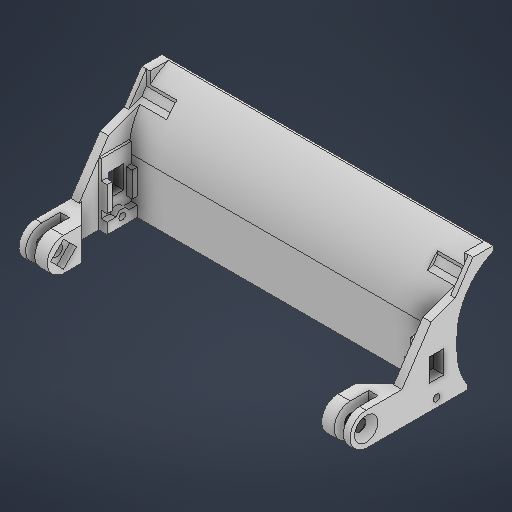
# Autodesk Inventor part: body-main
Saved by Autodesk Inventor 2025 (Build 290162000, 162)
## iProperties
Created: 2025-03-21
Part Number: body-main
Material: Všeobecné
Document SubType Name: Modeling
Designer: Simak
Density: 1 g/cm^3
Appearance: Výchozí
Author: Simak
Autodesk Inventor part; units mm, degrees
ref_plane "YZ Plane" through (0, 0, 0) normal (1, 0, 0) x (0, 1, 0)
ref_plane "XZ Plane" through (0, 0, 0) normal (0, 1, 0) x (-1, 0, 0)
ref_plane "XY Plane" through (0, 0, 0) normal (0, 0, 1) x (1, 0, 0)
sketch "Náčrt1" plane through (0, 0, 0) normal (1, 0, 0) x (0, 1, 0)
  circle A0 centre (13.5, 0) radius 16.5 construction
  circle A1 centre (15.5, 0) radius 16.5 construction
  circle A2 centre (11.5, 0) radius 16.5 construction
  line L0 (15.5, 16.5) -> (11.5, 16.5) construction
  line L1 (15.5, -16.5) -> (11.5, -16.5) construction
  circle A3 centre (5, 45.139) radius 5
  line L2 (0, 0) -> (0, 45.139)
  line L3 (10, 34.353) -> (22.9651, 25.7096)
  line L4 (10, 34.353) -> (10, 45.139)
  line L5 (22.9651, 25.7096) -> (27.5, 13.25)
  line L6 (27.5, 13.25) -> (33.5, 13.25)
  line L7 (33.5, 13.25) -> (25.5777, 18.5315)
  line L8 (33.5, 13.25) -> (33.5, 7.1937)
  line L9 (29, 13.25) -> (27.0194, 14.5704)
  arc A4 (13.5, -17.8885) -> (15.5, 18) centre (15.5, 0) ccw
  arc A5 (11.5, 18) -> (13.5, -17.8885) centre (11.5, 0) ccw
  line L10 (15.5, 18) -> (11.5, 18)
  line L11 (1.5, 14.9666) -> (0, 14.9666)
  line L12 (33.5, 7.1937) -> (32, 7.1937)
  arc A6 (13.5, -19.4977) -> (15.5, 19.6) centre (15.5, 0) ccw
  arc A7 (11.5, 19.6) -> (13.5, -19.4977) centre (11.5, 0) ccw
  line L13 (11.5, 19.6) -> (15.5, 19.6)
  line L14 (21.6, 28.6) -> (0, 28.6) construction
  line L15 (0, 28.6) -> (0, 19.6)
  line L16 (0, 19.6) -> (21.6, 19.6)
  line L17 (21.6, 19.6) -> (21.6, 28.6) construction
  line L18 (35.6, 21.5) -> (34, 21.5) construction
  line L19 (34, 21.5) -> (34, -16) construction
  line L20 (34, -16) -> (35.6, -16) construction
  line L21 (35.6, -16) -> (35.6, 21.5) construction
  line L22 (35.6, 17.75) -> (34, 17.75) construction
  line L23 (33.2196, 14.55) -> (26.5242, 14.55) construction
  line L24 (10, 39.639) -> (0, 39.639)
  line L25 (10, 34.353) -> (9.85, 34.453)
  line L26 (9.85, 34.453) -> (9.85, 39.639)
  point P0 (26.3917, 16.2951)
  point P1 (33.5, 7.7563)
  point P2 (29.9429, 13.25)
  dimension "d0" = 33
  dimension "d1" = 2
  dimension "d2" = 2
  dimension "d3" = 13.5
  dimension "d4" = 10
  dimension "d5" = 45.139
  dimension "d6" = 10.786
  dimension "d8" = 123.69
  dimension "d10" = 13.25
  dimension "d11" = 33.5
  dimension "d12" = 6
  dimension "d16" = 1.5
  dimension "d17" = 36
  dimension "d18" = 36
  dimension "d19" = 1.5
  dimension "d20" = 1.5
  dimension "d21" = 1.6
  dimension "d23" = 9
  dimension "d24" = 21.6
  dimension "d25" = 0.5
  dimension "d26" = 1.6
  dimension "d27" = 37.5
  dimension "d28" = 3.75
  dimension "d29" = 20.5
  dimension "d30" = 3.2
  dimension "d41" = 5.5
  dimension "d45" = 9.85
  dimension "d86" = 70
  constraints: 54 end point, 17 point on circle, 11 point on line, 8 centre point, 8 perpendicular, 7 horizontal, 5 parallel, 5 tangent, 3 horizontal alignment, 3 vertical, 2 coincident, 2 collinear, 2 equal radius, 2 other
  measures "d0" diameter of A0
  measures "d1" distance of A0.centre A1.centre
  measures "d2" distance of A0.centre A2.centre
  measures "d3" distance of A0.centre L2.start
  measures "d4" diameter of A3
  measures "d5" vertical distance of A3.centre A0.centre
  measures "d6" vertical distance of A3.centre L3.start
  measures "d8" angle of L4 L3
  measures "d10" distance from line of A1.centre L6
  measures "d11" distance from line of L2 L6.end
  measures "d12" distance of L5.end L6.end
  measures "d16" distance of L5.end L9.start
  measures "d17" diameter of A4
  measures "d18" diameter of A5
  measures "d19" distance of L11.start L11.end
  measures "d20" distance of L8.end L12.end
  measures "d21" radial gap between concentric circles of A4 A6
  measures "d23" distance of L16.end L14.start
  measures "d24" distance of L14.start L14.end
  measures "d25" distance between parallel lines of L20 L1
  measures "d26" distance of L19.end L20.end
  measures "d27" distance of L20.end L18.start
  measures "d28" distance between parallel lines of L18 L22
  measures "d29" distance from line of L19 A0.centre
  measures "d30" distance between parallel lines of L22 L23
  measures "d41" distance from line of A3.centre L24
  measures "d45" distance between parallel lines of L2 L26
  measures "d86" angle of L6 L5
extrude "Vysunutí1" add sketch "Náčrt1" against normal blind 2.5 contours L24 L26 L25 L3 L5 A6 L13 L16 L2 | L16 A7 L2 | A7 L13 A6 L5 A4 L10 A5 L11 L2 | L8 A6 L6 | L9 L6 A4 L5 | A6 L8 L12 A4 L6
extrude "Vysunutí3" add sketch "Náčrt1" against normal blind 49.5 contours L16 A7 L2 | A7 L13 A6 L5 A4 L10 A5 L11 L2 | A6 L6 L9 L5 | L9 L6 A4 L5 | A6 L8 L12 A4 L6
extrude "Vysunutí4" cut sketch "Náčrt1" against normal blind 10.5 contours A6 L6 L9 L5
extrude "Vysunutí5" add sketch "Náčrt1" against normal blind 1.35 contours L7 L6 A6 L5 | A6 L6 L9 L5
sketch "Náčrt2" plane through (0, 0, 0) normal (1, 0, 0) x (0, 0, -1)
  circle A0 centre (-45.139, 5) radius 4.85
  line L0 (-46.7978, 0.4425) -> (-45.5821, 0)
  line L1 (-19.6, 0) -> (-39.639, 0) projected
  line L2 (-39.639, 0) -> (-45.5821, 0)
  line L3 (-39.639, 9.85) -> (-39.639, 0) projected
  line L4 (-39.639, 9.85) -> (-45.139, 9.85)
  line L5 (-45.139, 8.8891) -> (-49.0281, 5)
  line L6 (-49.0281, 5) -> (-45.139, 1.1109)
  line L7 (-45.139, 1.1109) -> (-41.2499, 5)
  line L8 (-41.2499, 5) -> (-45.139, 8.8891)
  line L9 (-45.139, 8.8891) -> (-45.139, 5) construction
  line L10 (-45.139, 5) -> (-41.2499, 5) construction
  line L11 (-45.139, 5) -> (-45.139, 1.1109) construction
  point P0 (0, 0)
  dimension "d42" = 9.7
  dimension "d44" = 20
  dimension "d47" = 5.5
  constraints: 20 end point, 5 equal length, 4 perpendicular, 2 point on circle, 2 tangent, 1 centre point, 1 coincident, 1 collinear, 1 vertical
  measures "d42" diameter of A0
  measures "d44" angle of L2 L0
  measures "d47" distance of L7.end L5.start
extrude "Vysunutí6" add sketch "Náčrt2" against normal blind 8.5 contours A0 | A0 L4 L3 L2 L0 | L8 L7 L6 L5
sketch "Náčrt3" plane through (0, 0, 0) normal (1, 0, 0) x (0, 0, -1)
  arc A0 (-45.139, 9.85) -> (-46.7978, 0.4425) centre (-45.139, 5) ccw construction
  point P0 (0, 0)
  constraints: 1 coincident
hole "Díra1" at (0, 5, 45.139) direction (-1, 0, 0) diameter 3.4 end through all countersink diameter 7 countersink angle 90
sketch "Náčrt4" plane through (-8.5, 0, 0) normal (-1, 0, 0) x (0, 0, 1)
  line L0 (45.139, 1.1109) -> (41.2499, 5) projected
  line L1 (41.2499, 5) -> (45.139, 8.8891) projected
  line L2 (45.139, 8.8891) -> (49.0281, 5) projected
  line L3 (49.0281, 5) -> (45.139, 1.1109) projected
  point P0 (0, 0)
extrude "Vysunutí7" cut sketch "Náčrt4" against normal blind 2
sketch "Náčrt5" plane through (-2.5, 9.85, 34.453) normal (0, 1, 0) x (1, 0, 0)
  line L0 (2.5, -15.536) -> (-6, -15.536) projected
  line L1 (0.5, -15.536) -> (0.5, -5.186)
  line L2 (0.7, -12.386) -> (0.7, -8.986) projected
  line L3 (0.5, -5.186) -> (-2.25, -5.186)
  line L4 (-2.25, -5.186) -> (-2.25, -15.536)
  line L5 (2.5, 0) -> (2.5, -10.686) projected
  line L6 (2.5, -10.686) -> (-6, -10.686) projected
  line L7 (-6, -10.686) -> (-6, -5.186) projected
  line L8 (-6, -5.186) -> (0, 0.814)
  line L9 (0, 0) -> (0, 8.7433) projected
  line L10 (0, -5.186) -> (-6, -5.186) projected
  line L11 (0, -5.186) -> (0, 0) projected
  point P0 (2.5, 34.453)
  dimension "d59" = 2
  dimension "d60" = 2.75
  dimension "d61" = 5.5
  dimension "d62" = 45
  constraints: 8 end point, 2 perpendicular, 2 point on line, 1 parallel
  measures "d59" distance between parallel lines of L5 L1
  measures "d60" distance of L1.end L3.end
  measures "d61" distance between parallel lines of L3 L6
  measures "d62" angle of L10 L8
extrude "Vysunutí8" add sketch "Náčrt5" against normal up to surface (9.85 mm away) contours L10 L8 L9 L11 L3
extrude "Vysunutí9" cut sketch "Náčrt5" against normal through all contours L0 L4 L6 L1 | L6 L4 L3 L1
sketch "Náčrt6" plane through (-2.5, 0, 0) normal (-1, 0, 0) x (0, 0, 1)
  line L0 (19.6, 21.6) -> (28.6, 21.6) projected
  line L1 (28.6, 21.6) -> (28.6, 0) projected
  line L2 (19.6, 0) -> (19.6, 21.6) projected
  line L3 (19.6, 0) -> (33.639, 0) projected
  circle A0 centre (24.1, 2.54) radius 1
  line L4 (22.9, 13.2) -> (25.3, 13.2)
  line L5 (25.3, 13.2) -> (25.3, 8.4)
  line L6 (25.3, 8.4) -> (22.9, 8.4)
  line L7 (22.9, 8.4) -> (22.9, 13.2)
  line L8 (21.9, 14.2) -> (26.3, 14.2)
  line L9 (26.3, 14.2) -> (26.3, 7.4)
  line L10 (26.3, 7.4) -> (21.9, 7.4)
  line L11 (21.9, 7.4) -> (21.9, 14.2)
  line L12 (34.453, 9.85) -> (25.7096, 22.9651) projected
  line L13 (19.6, 18.85) -> (28.6, 18.85)
  point P0 (0, 0)
  point P1 (24.1, 21.6)
  point P2 (24.1, 13.2)
  point P3 (28.453, 18.85)
  point P4 (28.6, 18.6295)
  dimension "d67" = 2.54
  dimension "d68" = 2
  dimension "d69" = 2.4
  dimension "d70" = 4.8
  dimension "d71" = 8.4
  dimension "d72" = 1
  dimension "d77" = 2.75
  constraints: 18 end point, 4 parallel, 2 horizontal, 2 midpoint, 2 perpendicular, 2 point on line, 2 vertical alignment, 1 centre point, 3 other
  measures "d67" distance from line of L3 A0.centre
  measures "d68" diameter of A0
  measures "d69" distance of L4.start L4.end
  measures "d70" distance of L4.end L5.end
  measures "d71" distance between parallel lines of L3 L6
  measures "d72" distance between parallel lines of L7 L11
  measures "d77" distance between parallel lines of L0 L13
extrude "Vysunutí10" add sketch "Náčrt6" along normal blind 2.5 contours L13 L12 L1 L3 L2
extrude "Vysunutí11" cut sketch "Náčrt6" against normal through all contours A0 | L4 L5 L6 L7 | L8 L9 L10 L11
sketch "Náčrt7" plane through (-5, 0, 0) normal (-1, 0, 0) x (0, 0, 1)
  line L0 (19.6, 0) -> (19.6, 15.5) projected
  line L1 (19.6, 3.25) -> (28.6, 3.25)
  line L2 (28.6, 0) -> (28.6, 18.6295) projected
  line L3 (28.6, 5.5) -> (27.1, 5.5)
  line L4 (27.1, 5.5) -> (27.1, 13)
  line L5 (27.1, 13) -> (28.6, 13)
  line L6 (19.6, 13) -> (21.1, 13)
  line L7 (21.1, 13) -> (21.1, 5.5)
  line L8 (21.1, 5.5) -> (19.6, 5.5)
  circle A0 centre (24.1, 2.54) radius 1 projected
  line L9 (19.6, 0) -> (28.6, 0) projected
  circle A1 centre (24.1, 2.54) radius 2
  line L10 (19.6, 18.85) -> (19.6, 15.5) projected
  line L11 (19.6, 0) -> (19.6, 15.5) projected
  line L12 (19.6, 0) -> (28.6, 0) projected
  line L13 (28.6, 0) -> (28.6, 18.6295) projected
  line L14 (28.453, 18.85) -> (19.6, 18.85) projected
  line L15 (21.9, 14.2) -> (26.3, 14.2) projected
  line L16 (26.3, 14.2) -> (26.3, 7.4) projected
  line L17 (26.3, 7.4) -> (21.9, 7.4) projected
  line L18 (21.9, 7.4) -> (21.9, 14.2) projected
  circle A2 centre (24.1, 2.54) radius 1 projected
  line L19 (28.6, 18.6295) -> (28.453, 18.85) projected
  point P0 (0, 0)
  point P1 (28.6, 18.85)
  point P2 (28.6, 18.85)
  point P3 (22.2303, 3.25)
  point P4 (25.9697, 3.25)
  dimension "d78" = 1.5
  dimension "d79" = 7.5
  dimension "d80" = 13
  dimension "d82" = 3.25
  dimension "d83" = 1
  constraints: 14 end point, 8 point on line, 4 perpendicular, 2 equal length, 2 horizontal, 1 centre point, 1 horizontal alignment
  measures "d78" distance of L4.end L5.end
  measures "d79" distance of L6.end L7.end
  measures "d80" distance between parallel lines of L9 L6
  measures "d82" distance between parallel lines of L9 L1
  measures "d83" radial gap between concentric circles of A0 A1
extrude "Vysunutí12" cut sketch "Náčrt7" against normal blind 1.75 contours L0 L8 L7 L6 L10 L14 L19 L2 L5 L4 L3 L1 A1
mirror "Zrcadlit1" about plane through (-49.5, 16.75, 13.3969) normal (-1, 0, 0)
equation "\"d2\" = d1"
equation "\"d18\" = d17"
